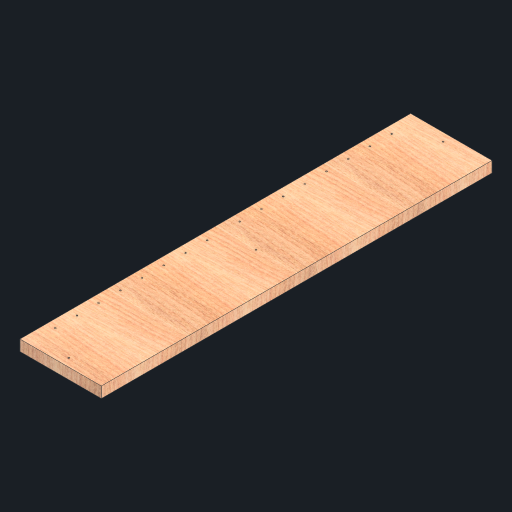
# Autodesk Inventor part: Side Panel
Saved by Autodesk Inventor 2024.2 (Build 282272000, 272)
## iProperties
Created: 2025-06-28
Part Number: Side Panel
Material: Wood (Birch)
Document SubType Name: Modeling
Designer: Bryan
Density: 0.55 g/cm^3
Appearance: Birch - Natural Polished
Mass: 2431.38 g
Surface Area: 4090.28 cm^2
Volume: 4420.69 cm^3
Author: Bryan
Autodesk Inventor part; units mm, degrees
ref_plane "YZ Plane" through (0, 0, 0) normal (1, 0, 0) x (0, 1, 0)
ref_plane "XZ Plane" through (0, 0, 0) normal (0, 1, 0) x (-1, 0, 0)
ref_plane "XY Plane" through (0, 0, 0) normal (0, 0, 1) x (1, 0, 0)
sketch "Sketch1" plane through (0, 0, 0) normal (0, 1, 0) x (-1, 0, 0)
  line L0 (0, 0) -> (190.5, 0)
  line L1 (190.5, 0) -> (190.5, -914.4)
  line L2 (190.5, -914.4) -> (0, -914.4)
  line L3 (0, -914.4) -> (0, 0)
  dimension "d0" = 190.5
  dimension "d1" = 914.4
  constraints: 8 end point, 2 parallel, 1 horizontal, 1 perpendicular
  measures "d0" distance of L1.end L2.end
  measures "d1" distance of L0.end L1.end
extrude "Extrusion1" add sketch "Sketch1" along normal blind 25.4
sketch "Sketch2" plane through (0, 25.4, 0) normal (0, 1, 0) x (1, 0, 0)
  line L0 (0, 914.4) -> (-190.5, 914.4) construction
  line L1 (-190.5, 914.4) -> (-190.5, 0) construction
  line L2 (-190.5, 0) -> (0, 0) construction
  line L3 (0, 0) -> (0, 914.4) construction
  line L4 (-152.4, 876.3) -> (0, 876.3) construction
  line L5 (0, 38.1) -> (-152.4, 38.1) construction
  line L6 (-152.4, 38.1) -> (-152.4, 876.3) construction
  line L7 (-152.4, 476.25) -> (0, 476.25) construction
  line L8 (0, 438.15) -> (-152.4, 438.15) construction
  line L9 (-76.2, 476.25) -> (-76.2, 438.15) construction
  line L10 (0, 914.4) -> (0, 876.3) construction
  line L11 (0, 895.35) -> (-190.5, 895.35) construction
  line L12 (-152.4, 876.3) -> (-190.5, 876.3) construction
  line L13 (-152.4, 457.2) -> (-190.5, 457.2) construction
  line L14 (-171.45, 876.3) -> (-171.45, 457.2) construction
  line L15 (0, 457.2) -> (-76.2, 457.2) construction
  line L16 (-76.2, 457.2) -> (-152.4, 457.2) construction
  circle A0 centre (-50.8, 895.35) radius 1.5875
  circle A1 centre (-95.25, 895.35) radius 1.5875
  circle A2 centre (-171.45, 850.9) radius 1.5875
  circle A3 centre (-171.45, 800.1) radius 1.5875
  circle A4 centre (-171.45, 749.3) radius 1.5875
  circle A5 centre (-171.45, 698.5) radius 1.5875
  circle A6 centre (-171.45, 647.7) radius 1.5875
  circle A7 centre (-171.45, 596.9) radius 1.5875
  circle A8 centre (-171.45, 546.1) radius 1.5875
  circle A9 centre (-171.45, 495.3) radius 1.5875
  circle A10 centre (-50.8, 457.2) radius 1.5875
  circle A11 centre (-95.25, 457.2) radius 1.5875
  circle A12 centre (-50.8, 19.05) radius 1.5875
  circle A13 centre (-95.25, 19.05) radius 1.5875
  circle A14 centre (-171.45, 63.5) radius 1.5875
  circle A15 centre (-171.45, 114.3) radius 1.5875
  circle A16 centre (-171.45, 165.1) radius 1.5875
  circle A17 centre (-171.45, 215.9) radius 1.5875
  circle A18 centre (-171.45, 266.7) radius 1.5875
  circle A19 centre (-171.45, 317.5) radius 1.5875
  circle A20 centre (-171.45, 368.3) radius 1.5875
  circle A21 centre (-171.45, 419.1) radius 1.5875
  dimension "d4" = 38.1
  dimension "d5" = 38.1
  dimension "d6" = 38.1
  dimension "d7" = 50.8
  dimension "d8" = 3.175
  dimension "d9" = 3.175
  dimension "d10" = 3.175
  dimension "d11" = 25.4
  dimension "d14" = 50.8
  constraints: 26 end point, 22 centre point, 12 point on line, 10 midpoint, 10 symmetric about line, 5 horizontal, 2 coincident, 2 equal radius, 2 vertical, 2 vertical alignment, 1 horizontal alignment, 25 other
  measures "d4" distance between parallel lines of L0 L4
  measures "d5" distance between parallel lines of L1 L6
  measures "d6" distance between parallel lines of L8 L7
  measures "d7" distance from line of L10 point (-50.8, 895.35)
  measures "d8" diameter of A0
  measures "d9" diameter of A1
  measures "d10" diameter of A2
  measures "d11" distance from line of A2.centre L12
  measures "d14" distance of A2.centre A3.centre
extrude "Extrusion2" cut sketch "Sketch2" against normal through all contours A1 | A2 | A3 | A4 | A5 | A6 | A7 | A8 | A9 | A11 | A13 | A14 | A15 | A16 | A17 | A18 | A19 | A20 | A21
equation "\"d5\" = d4"
equation "\"d6\" = d4"
body "Solid1"
